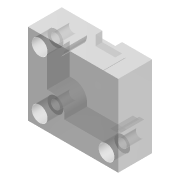
# Autodesk Inventor part: case_top
Saved by Autodesk Inventor 2015 SP1 (Build 190203100, 203)
## iProperties
Created: 2015-12-01
Part Number: case_top
Material: Polycarbonate, Clear
Document SubType Name: Modeling
Designer: User
Density: 1.2 g/cm^3
Appearance: Polycarbonate - Clear
Mass: 15.4954 g
Surface Area: 70.56 cm^2
Volume: 12.9128 cm^3
Author: User
Autodesk Inventor part; units mm, degrees
ref_plane "YZ Plane" through (0, 0, 0) normal (1, 0, 0) x (0, 1, 0)
ref_plane "XZ Plane" through (0, 0, 0) normal (0, 1, 0) x (-1, 0, 0)
ref_plane "XY Plane" through (0, 0, 0) normal (0, 0, 1) x (1, 0, 0)
sketch "Эскиз1" plane through (0, 0, 0) normal (0, 1, 0) x (-1, 0, 0)
  line L0 (18, -16) -> (-18, -16)
  line L1 (-18, -16) -> (-18, 16)
  line L2 (-18, 16) -> (18, 16)
  line L3 (18, 16) -> (18, -16)
  line L4 (0, -25.2) -> (0, 25.2) projected
  line L5 (28, 0) -> (-28, 0) projected
  line L6 (14.82, -12.82) -> (-14.82, -12.82)
  line L7 (-14.82, -12.82) -> (-14.82, 12.82)
  line L8 (-14.82, 12.82) -> (14.82, 12.82)
  line L9 (14.82, 12.82) -> (14.82, -12.82)
  circle A0 centre (14.82, -12.82) radius 2
  circle A1 centre (14.82, 12.82) radius 2
  circle A2 centre (-14.82, 12.82) radius 2
  circle A3 centre (-14.82, -12.82) radius 2
  arc A4 (14.82, -6.82) -> (8.82, -12.82) centre (14.82, -12.82) ccw
  arc A5 (-8.82, -12.82) -> (-14.82, -6.82) centre (-14.82, -12.82) ccw
  arc A6 (8.82, 12.82) -> (14.82, 6.82) centre (14.82, 12.82) ccw
  arc A7 (-14.82, 6.82) -> (-8.82, 12.82) centre (-14.82, 12.82) ccw
  line L10 (20, -18) -> (-20, -18)
  line L11 (-20, -18) -> (-20, 18)
  line L12 (-20, 18) -> (20, 18)
  line L13 (20, 18) -> (20, -18)
  line L14 (-8.82, -12.82) -> (-8.82, -16)
  line L15 (8.82, -12.82) -> (8.82, -16)
  line L16 (14.82, -6.82) -> (18, -6.82)
  line L17 (14.82, 6.82) -> (18, 6.82)
  line L18 (8.82, 12.82) -> (8.82, 16)
  line L19 (-14.82, -6.82) -> (-20, -6.82)
  line L20 (-14.82, 6.82) -> (-20, 6.82)
  line L21 (-8.82, 12.82) -> (-8.82, 18)
  line L22 (-18, -6.82) -> (-18, 6.82)
  line L23 (8.82, 16) -> (-8.82, 16)
  line L24 (2, 13.6) -> (-6.7, 13.6)
  line L25 (-6.7, 13.6) -> (-6.7, 18)
  line L26 (3.5, 16) -> (3.5, 12.6)
  line L27 (3.5, 12.6) -> (-8.2, 12.6)
  line L28 (-8.2, 12.6) -> (-8.2, 16)
  line L29 (2, 13.6) -> (2, 18)
  circle A8 centre (-14.82, -12.82) radius 3.5
  circle A9 centre (14.82, -12.82) radius 3.5
  circle A10 centre (14.82, 12.82) radius 3.5
  circle A11 centre (-14.82, 12.82) radius 4
  line L30 (18, 6.82) -> (16.5, 6.82)
  line L31 (16.5, 6.82) -> (16.5, -6.82)
  line L32 (16.5, -6.82) -> (18, -6.82)
  line L33 (18, -6.82) -> (18, 6.82)
  line L34 (8.82, 16) -> (3.5, 16)
  line L35 (3.5, 16) -> (3.5, 14.5)
  line L36 (3.5, 14.5) -> (8.82, 14.5)
  line L37 (8.82, 14.5) -> (8.82, 16)
  line L38 (-8.2, 16) -> (-8.82, 16)
  line L39 (-8.82, 16) -> (-8.82, 14.5)
  line L40 (-8.82, 14.5) -> (-8.2, 14.5)
  line L41 (-8.2, 14.5) -> (-8.2, 16)
  line L42 (-18, 6.82) -> (-16.5, 6.82)
  line L43 (-16.5, 6.82) -> (-16.5, -6.82)
  line L44 (-16.5, -6.82) -> (-18, -6.82)
  line L45 (-18, -6.82) -> (-18, 6.82)
  line L46 (8.82, -16) -> (-8.82, -16)
  line L47 (-8.82, -16) -> (-8.82, -14.41)
  line L48 (8.82, -14.41) -> (8.82, -16)
  line L49 (8.82, -16) -> (-8.82, -16)
  line L50 (-8.82, -16) -> (-8.82, -14.5)
  line L51 (-8.82, -14.5) -> (8.82, -14.5)
  line L52 (8.82, -14.5) -> (8.82, -16)
  line L53 (-11.5034, -7.82) -> (-14.32, -7.82)
  line L54 (-14.32, -7.82) -> (-14.32, -6.8409)
  point P0 (0, 0)
  point P1 (-13.034, 10.913)
  dimension "d0" = 36
  dimension "d1" = 32
  dimension "d2" = 3.18
  dimension "d3" = 3.18
  dimension "d4" = 3.18
  dimension "d5" = 3.18
  dimension "d6" = 4
  dimension "d7" = 4
  dimension "d8" = 4
  dimension "d9" = 4
  dimension "d10" = 12
  dimension "d11" = 12
  dimension "d12" = 12
  dimension "d13" = 12
  dimension "d22" = 4.966
  dimension "d23" = 5.087
  dimension "d26" = 2
  dimension "d27" = 2
  dimension "d28" = 2
  dimension "d29" = 2
  dimension "d40" = 11.3
  dimension "d41" = 2.4
  dimension "d43" = 1
  dimension "d44" = 1.5
  dimension "d45" = 1.5
  dimension "d46" = 16
  dimension "d49" = 7
  dimension "d50" = 7
  dimension "d51" = 7
  dimension "d52" = 8
  dimension "d63" = 1.5
  dimension "d64" = 1.5
  dimension "d65" = 1.5
  dimension "d66" = 1.5
  dimension "d67" = 1.5
  dimension "d68" = 0.5
  dimension "d69" = 5
  constraints: 106 end point, 31 point on line, 21 perpendicular, 17 parallel, 12 centre point, 12 coincident, 11 horizontal, 10 point on circle, 3 tangent, 1 midpoint, 1 vertical, 2 other
  measures "d0" distance of L0.start L0.end
  measures "d1" distance of L0.end L1.end
  measures "d2" distance between parallel lines of L3 L9
  measures "d3" distance between parallel lines of L2 L8
  measures "d4" distance between parallel lines of L1 L7
  measures "d5" distance between parallel lines of L0 L6
  measures "d6" diameter of A0
  measures "d7" diameter of A1
  measures "d8" diameter of A2
  measures "d9" diameter of A3
  measures "d10" diameter of A4
  measures "d11" diameter of A5
  measures "d12" diameter of A6
  measures "d13" diameter of A7
  measures "d22" distance from line of L1 point (-13.034, 10.913)
  measures "d23" distance from line of L2 point (-13.034, 10.913)
  measures "d26" distance between parallel lines of L10 L0
  measures "d27" distance between parallel lines of L13 L3
  measures "d28" distance between parallel lines of L2 L12
  measures "d29" distance between parallel lines of L11 L1
  measures "d40" distance between parallel lines of L1 L25
  measures "d41" distance between parallel lines of L23 L24
  measures "d43" distance between parallel lines of L27 L24
  measures "d44" distance between parallel lines of L25 L28
  measures "d45" distance between parallel lines of L26 L29
  measures "d46" distance between parallel lines of L3 L29
  measures "d49" diameter of A8
  measures "d50" diameter of A9
  measures "d51" diameter of A10
  measures "d52" diameter of A11
  measures "d63" distance between parallel lines of L33 L31
  measures "d64" distance between parallel lines of L2 L36
  measures "d65" distance between parallel lines of L2 L40
  measures "d66" distance between parallel lines of L1 L43
  measures "d67" distance between parallel lines of L46 L51
  measures "d68" distance between parallel lines of L7 L54
  measures "d69" distance between parallel lines of L6 L53
extrude "Выдавливание1" add sketch "Эскиз1" along normal blind 15 contours L3 A9 L5 L13 L10 L4 L0 | L0 A9 L3 | A9 L0 | L0 A9 L6 A0 L9 L3 | L3 A9 | L0 L15 L6 A9 | A9 L9 L16 L3 | L0 L4 L51 L15 | A9 L9 A0 L6 | L6 A4 L9 A9 | L16 L31 L5 L3 | L4 L10 L11 L19 L1 A8 L0 | L0 L14 L51 L4 | A0 L9 L6 | L6 L9 A0 | L5 L31 L17 L3 | L3 A10 L2 L29 L12 L13 L5 | L0 A8 L6 L14 | L17 L9 A10 L3 | A8 L0 | L0 A8 L1 L7 A3 L6 | L6 A8 L7 A5 L54 L53 | A10 L9 A1 L8 L2 L3 | L3 A10 | A6 L8 A10 L9 | L0 L1 A8 | L6 A3 L7 A8 | L11 L5 L1 L19 | L27 L28 L8 L4 | L4 L8 L26 L27 | L53 L54 A5 | A10 L2 L3 | A10 L8 A1 L9 | L29 L2 L4 L12 | L18 L2 A10 L8 | L8 L26 L36 L18 | A8 L1 | A3 L7 L6 | L6 L7 A3 | A8 L1 L19 L7 | L11 L20 L1 L5 | L1 L5 L43 L19 | L8 L28 L2 L25 L24 L4 | L4 L24 L29 L2 L26 L8 | L5 L1 L20 L43 | L20 L1 A11 L7 | L7 A11 L8 A7 | L2 A10 | A1 L8 L9 | L9 L8 A1 | L4 L2 L25 L12 | L29 L24 L4 L2 | L36 L26 L2 L18 | L11 L12 L21 L2 A11 L1 L20 | L24 L25 L2 L4 | L8 L21 L40 L28 | A11 L1 L2 L8 A2 L7 | L7 A2 L8 A11 | L8 A11 L2 L21 | L25 L2 L21 L12 | L40 L21 L2 L28 | A2 L8 L7 | L7 L8 A2 | A11 L1 | L1 L2 A11 | L2 A11
extrude "Выдавливание2" add sketch "Эскиз1" along normal blind 5 contours L3 A9 L5 L13 L10 L4 L0 | L0 A9 L3 | A9 L0 | L0 A9 L6 A0 L9 L3 | L3 A9 | L0 L15 L6 A9 | A9 L9 L16 L3 | L0 L4 L51 L15 | A9 L9 A0 L6 | L6 A4 L9 A9 | L16 L31 L5 L3 | L4 L10 L11 L19 L1 A8 L0 | L0 L14 L51 L4 | L51 L4 L6 L15 | A0 L9 L6 | L6 L9 A0 | L6 L4 L5 L9 A4 | L5 L31 L17 L3 | L3 A10 L2 L29 L12 L13 L5 | L16 L9 L5 L31 | L0 A8 L6 L14 | L51 L14 L6 L4 | L6 A5 L7 L5 L4 | L17 L9 A10 L3 | L5 L9 L17 L31 | L5 L4 L27 L26 L8 A6 L9 | A8 L0 | L0 A8 L1 L7 A3 L6 | L5 L7 A7 L8 L28 L27 L4 | L6 A8 L7 A5 L54 L53 | A10 L9 A1 L8 L2 L3 | L3 A10 | A6 L8 A10 L9 | L0 L1 A8 | L6 A3 L7 A8 | L11 L5 L1 L19 | L27 L28 L8 L4 | L4 L8 L26 L27 | L7 L19 L43 L5 | L5 L43 L20 L7 | L53 L54 A5 | A10 L2 L3 | A10 L8 A1 L9 | L29 L2 L4 L12 | L18 L2 A10 L8 | L8 L26 L36 L18 | A8 L1 | A3 L7 L6 | L6 L7 A3 | A8 L1 L19 L7 | L11 L20 L1 L5 | L1 L5 L43 L19 | L8 L28 L2 L25 L24 L4 | L4 L24 L29 L2 L26 L8 | L5 L1 L20 L43 | L20 L1 A11 L7 | L7 A11 L8 A7 | L2 A10 | L4 L2 L25 L12 | L29 L24 L4 L2 | L36 L26 L2 L18 | L11 L12 L21 L2 A11 L1 L20 | L24 L25 L2 L4 | L8 L21 L40 L28 | A11 L1 L2 L8 A2 L7 | L7 A2 L8 A11 | L8 A11 L2 L21 | L25 L2 L21 L12 | L40 L21 L2 L28 | A2 L8 L7 | L7 L8 A2 | A11 L1 | L1 L2 A11 | L2 A11
sketch "Эскиз2" plane through (0, 15, 0) normal (0, 1, 0) x (1, 0, 0)
  circle A0 centre (-14.82, -12.82) radius 2 projected
  circle A1 centre (14.82, -12.82) radius 2 projected
  circle A2 centre (14.82, 12.82) radius 2 projected
  circle A3 centre (-14.82, 12.82) radius 2 projected
  point P0 (0, 0)
extrude "Выдавливание3" cut sketch "Эскиз2" against normal up to next contours A0 | A2 | A3
extrude "Выдавливание5" cut sketch "Эскиз1" along normal blind 7 contours A9 L0 | L0 A9 L6 A0 L9 L3 | L3 A9 | A9 L9 A0 L6 | A8 L0 | L0 A8 L1 L7 A3 L6 | A10 L9 A1 L8 L2 L3 | L3 A10 | L6 A3 L7 A8 | A10 L8 A1 L9 | A8 L1 | L2 A10
sketch "Эскиз3" plane through (0, 15, 0) normal (0, 1, 0) x (1, 0, 0)
  line L0 (-20, -18) -> (20, -18) projected
  line L1 (-2, -13.6) -> (-2, -18) projected
  line L2 (-2, -13.6) -> (6.7, -13.6) projected
  line L3 (6.7, -13.6) -> (6.7, -18) projected
  point P0 (0, 0)
extrude "Выдавливание6" cut sketch "Эскиз3" against normal blind 3
sketch "Эскиз4" plane through (0, 15, 0) normal (0, 1, 0) x (1, 0, 0)
  line L0 (11.5034, 7.82) -> (14.32, 7.82) projected
  line L1 (14.32, 7.82) -> (14.32, 6.8409) projected
  arc A0 (8.82, 12.82) -> (14.82, 6.82) centre (14.82, 12.82) ccw projected
  point P0 (0, 0)
extrude "Выдавливание7" cut sketch "Эскиз4" against normal up to surface (10 mm away)
